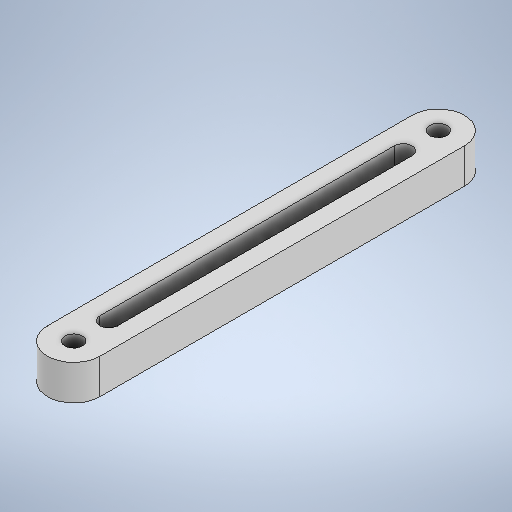
# Autodesk Inventor part: 6P-017
Saved by Autodesk Inventor 2025.2 (Build 292293000, 293)
## iProperties
Created: 2025-01-15
Part Number: 6P-017
Material: Generic
Document SubType Name: Modeling
Designer: Sameer Alhindi
Density: 1 g/cm^3
Appearance: Default
Author: Sameer Alhindi
Autodesk Inventor part; units mm, degrees
ref_plane "YZ Plane" through (0, 0, 0) normal (1, 0, 0) x (0, 1, 0)
ref_plane "XZ Plane" through (0, 0, 0) normal (0, 1, 0) x (-1, 0, 0)
ref_plane "XY Plane" through (0, 0, 0) normal (0, 0, 1) x (1, 0, 0)
sketch "Sketch1" plane through (0, 0, 0) normal (0, 1, 0) x (-1, 0, 0)
  line L0 (0, 0) -> (0, -52) construction
  line L1 (-3.75, 0) -> (-3.75, -52)
  line L2 (3.75, -52) -> (3.75, 0)
  arc A0 (3.75, 0) -> (-3.75, 0) centre (0, 0) ccw
  arc A1 (-3.75, -52) -> (3.75, -52) centre (0, -52) ccw
  circle A2 centre (0, 0) radius 1.25
  circle A3 centre (0, -52) radius 1.25
  line L3 (0, -5) -> (0, -47) construction
  line L4 (-1.25, -5) -> (-1.25, -47)
  line L5 (1.25, -47) -> (1.25, -5)
  arc A4 (1.25, -5) -> (-1.25, -5) centre (0, -5) ccw
  arc A5 (-1.25, -47) -> (1.25, -47) centre (0, -47) ccw
  point P0 (0, -26)
  point P1 (0, -26)
  point P2 (0, -48.25)
  dimension "d0" = 52
  dimension "d1" = 7.5
  dimension "d2" = 2.5
  dimension "d3" = 2.5
  dimension "d4" = 26
  dimension "d7" = 3.75
  dimension "d8" = 2.5
  constraints: 16 end point, 9 point on circle, 8 tangent, 6 centre point, 2 coincident, 2 midpoint, 2 parallel, 2 point on line, 1 vertical
  measures "d0" distance of L0.start L0.end
  measures "d1" diameter of A1
  measures "d2" diameter of A2
  measures "d3" diameter of A3
  measures "d4" distance of point (0, -26) L0.start
  measures "d7" distance of point (0, -48.25) L0.end
  measures "d8" distance between parallel lines of L4 L5
extrude "Extrusion1" add sketch "Sketch1" along normal blind 5
equation "\"d4\" = 0.5 * d0"
body "Solid1"
